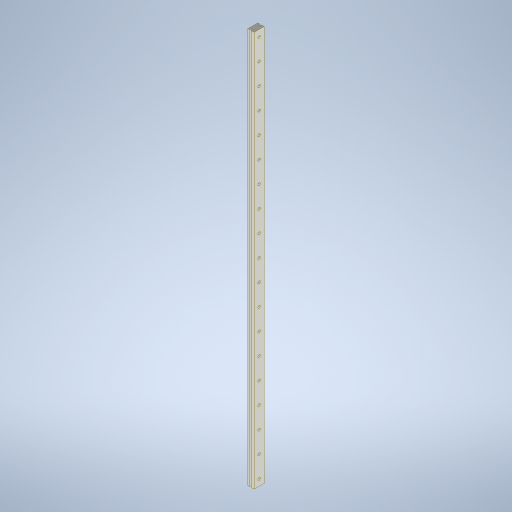
# Autodesk Inventor part: Trilho
Saved by Autodesk Inventor 2023 (Build 270158000, 158)
## iProperties
Created: 2023-04-01
Part Number: Trilho
Material: Aço inoxidável
Document SubType Name: Sheet Metal
Designer: Mateus PC
Density: 8 g/cm^3
Sheet Metal Rule: Default_mm
Appearance: Prata
Author: Mateus PC
Autodesk Inventor part; units mm, degrees
ref_plane "YZ Plane" through (0, 0, 0) normal (1, 0, 0) x (0, 1, 0)
ref_plane "XZ Plane" through (0, 0, 0) normal (0, 1, 0) x (-1, 0, 0)
ref_plane "XY Plane" through (0, 0, 0) normal (0, 0, 1) x (1, 0, 0)
sketch "Esboço1" plane through (0, 0, 0) normal (0, 1, 0) x (-1, 0, 0)
  line L0 (0, 0) -> (3.5, 0)
  line L1 (4, -2) -> (5, -2)
  line L2 (5.5, 0) -> (7.5, 0)
  line L3 (7.5, 0) -> (7.5, -12)
  line L4 (7.5, -12) -> (5.5, -12)
  line L5 (5, -10) -> (4, -10)
  line L6 (3.5, -12) -> (0, -12)
  line L7 (0, -12) -> (0, 0)
  line L8 (5.5, 0) -> (5, -2)
  line L9 (3.5, 0) -> (4, -2)
  line L10 (5, -10) -> (5.5, -12)
  line L11 (3.5, -12) -> (4, -10)
  dimension "d0" = 7.5
  dimension "d1" = 12
  dimension "d2" = 8
  dimension "d3" = 1
  dimension "d4" = 3.5
  dimension "d5" = 0.5
  constraints: 24 end point, 4 point on line, 3 equal length, 3 perpendicular, 1 horizontal, 1 parallel
  measures "d0" distance of L0.start L2.end
  measures "d1" distance of L6.end L0.start
  measures "d2" distance of L1.end L5.start
  measures "d3" distance of L1.start L1.end
  measures "d4" distance of L0.start L0.end
  measures "d5" horizontal distance of L2.start L1.end
extrude "Extrusão1" add sketch "Esboço1" along normal blind 469
sketch "Esboço2" plane through (-7.5, 0, -12) normal (-1, 0, 0) x (0, 0, 1)
  line L0 (0, 0) -> (0, 469) projected
  line L1 (0, 0) -> (12, 0) projected
  line L2 (12, 0) -> (12, 469) projected
  line L3 (12, 0) -> (0, 0) projected
  point P0 (6, 7.7)
  point P1 (6, 32.9)
  point P2 (6, 58.1)
  point P3 (6, 83.3)
  point P4 (6, 108.5)
  point P5 (6, 133.7)
  point P6 (6, 158.9)
  point P7 (6, 184.1)
  point P8 (6, 209.3)
  point P9 (6, 234.5)
  point P10 (6, 259.7)
  point P11 (6, 284.9)
  point P12 (6, 310.1)
  point P13 (6, 335.3)
  point P14 (6, 360.5)
  point P15 (6, 385.7)
  point P16 (6, 410.9)
  point P17 (6, 436.1)
  point P18 (6, 0)
  point P19 (6, 461.3)
  point P20 (6, 0)
  dimension "d10" = 25.2
  dimension "d18" = 6
  dimension "d27" = 453.6
  dimension "d28" = 469
  dimension "d29" = 7.7
  constraints: 2 midpoint, 1 vertical, 18 other
  measures "d10" distance of point (6, 7.7) point (6, 32.9)
  measures "d18" distance from line of L2 point (6, 7.7)
  measures "d27" distance of point (6, 7.7) point (6, 461.3)
  measures "d28" distance of L1.end L2.end
  measures "d29" distance of point (6, 0) point (6, 7.7)
hole "Furo1" at (-7.5, 7.7, -6) at (-7.5, 32.9, -6) at (-7.5, 58.1, -6) at (-7.5, 83.3, -6) at (-7.5, 108.5, -6) at (-7.5, 133.7, -6) at (-7.5, 158.9, -6) at (-7.5, 184.1, -6) at (-7.5, 209.3, -6) at (-7.5, 234.5, -6) at (-7.5, 259.7, -6) at (-7.5, 284.9, -6) at (-7.5, 310.1, -6) at (-7.5, 335.3, -6) at (-7.5, 360.5, -6) at (-7.5, 385.7, -6) at (-7.5, 410.9, -6) at (-7.5, 436.1, -6) at (-7.5, 461.3, -6) direction (1, 0, 0) diameter 3 depth 7.5 counterbore diameter 4 counterbore depth 2
equation "\"d29\" = -0.5 * d27 + 0.5 * d28"
equation "\"d24\" = Espessura"
equation "\"Raio_vergadura\" = Espessura"
equation "\"Largura_alívio_de_vergadura\" = Espessura"
equation "\"Profundidade_alívio_de_vergadura\" = 0.5 * Espessura"
equation "\"Tamanho_alívio_de_dobra\" = 4 * Espessura"
equation "\"Remanescente_mínimo\" = 2 * Espessura"
equation "\"Raiodetransição\" = Raio_vergadura"
equation "\"Tamanho_de_raio_de_Jacobi\" = Raio_vergadura"
equation "\"TamanhoFolga\" = Espessura"
equation "\"Espessura\" = 0.5"
